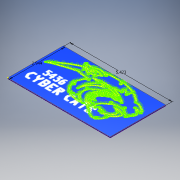
# Autodesk Inventor part: CyberCat Logo 1-27-2017
Saved by Autodesk Inventor 2016 SP2 (Build 200236200, 236)
## iProperties
Created: 2017-01-28
Part Number: CyberCat Logo 1-27-2017
Material: Generic
Document SubType Name: Modeling
Designer: CAD
Density: 1 g/cm^3
Appearance: Default
Author: CAD
Autodesk Inventor part; units mm, degrees
(part 1 of 3)
ref_plane "YZ Plane" through (0, 0, 0) normal (1, 0, 0) x (0, 1, 0)
ref_plane "XZ Plane" through (0, 0, 0) normal (0, 1, 0) x (-1, 0, 0)
ref_plane "XY Plane" through (0, 0, 0) normal (0, 0, 1) x (1, 0, 0)
sketch "Sketch5" plane through (0, 0, 0) normal (0, 1, 0) x (-1, 0, 0)
  line L0 (0, 0) -> (0, -74.7776)
  line L1 (0, -74.7776) -> (-137.7442, -74.7776)
  line L2 (-137.7442, -74.7776) -> (-137.7442, 0)
  line L3 (-137.7442, 0) -> (0, 0)
  dimension "d59" = 74.7776
  dimension "d60" = 137.7442
  constraints: 8 end point, 3 perpendicular, 1 vertical
  measures "d59" distance of L0.start L0.end
  measures "d60" distance of L0.end L1.end
extrude "Extrusion2" add sketch "Sketch5" along normal blind 0.7937
sketch "Sketch6" plane through (0, 0.7937, 0) normal (0, 1, 0) x (1, 0, 0)
  line L0 (137.7442, 74.7776) -> (0, 74.7776) projected
  line L1 (0, 74.7776) -> (137.7451, 74.7759) construction
  line L2 (137.7451, 74.7759) -> (137.7442, 0) construction
  line L3 (137.7442, 0) -> (-0.0009, 0.0017) construction
  line L4 (-0.0009, 0.0017) -> (0, 74.7776) construction
  point P0 (0, 0)
  constraints: 2 other
decal "Decal1"
sketch "Sketch7" plane through (0, 0.7937, 0) normal (0, 1, 0) x (1, 0, 0)
  circle A0 centre (6.8078, 44.1868) radius 1.651
  circle A1 centre (35.2483, 69.5859) radius 1.651
  circle A2 centre (41.5129, 60.1607) radius 1.651
  circle A3 centre (49.8624, 58.3881) radius 1.651
  circle A4 centre (44.4496, 66.9531) radius 1.651
  circle A5 centre (53.1196, 65.2289) radius 1.651
  circle A6 centre (57.1286, 60.9965) radius 1.651
  circle A7 centre (63.7205, 68.4202) radius 1.651
  circle A8 centre (83.2485, 68.8372) radius 1.651
  circle A9 centre (93.5061, 60.1607) radius 1.651
  circle A10 centre (99.5004, 60.1607) radius 1.651
  circle A11 centre (114.5732, 57.5147) radius 1.651
  circle A12 centre (130.6019, 48.3074) radius 1.651
  circle A13 centre (120.3092, 50.7732) radius 1.651
  circle A14 centre (127.1666, 41.9144) radius 1.651
  circle A15 centre (56.094, 53.7186) radius 1.651
  circle A16 centre (51.8293, 37.1588) radius 1.651
  circle A17 centre (59.035, 35.2533) radius 1.651
  circle A18 centre (64.8224, 41.5541) radius 1.651
  circle A19 centre (61.2211, 26.4773) radius 1.651
  circle A20 centre (65.5853, 26.8249) radius 1.651
  circle A21 centre (79.684, 21.2186) radius 1.651
  circle A22 centre (66.9848, 54.8596) radius 1.651
  circle A23 centre (78.8358, 51.8496) radius 1.651
  circle A24 centre (82.097, 53.5006) radius 1.651
  circle A25 centre (105.6651, 47.4221) radius 1.651
  circle A26 centre (97.355, 41.2731) radius 1.651
  circle A27 centre (84.8207, 32.3826) radius 1.651
  circle A28 centre (86.4717, 27.6903) radius 1.651
  arc A29 (94.6466, 25.5556) -> (93.8506, 25.9892) centre (95.008, 27.1666) ccw
  arc A30 (93.8506, 25.9892) -> (94.6466, 25.5556) centre (93.4892, 24.3783) ccw
  circle A31 centre (99.9904, 23.2455) radius 1.651
  circle A32 centre (104.8487, 13.4279) radius 1.651
  circle A33 centre (112.4853, 20.5125) radius 1.651
  circle A34 centre (113.5071, 44.1965) radius 1.651
  circle A35 centre (124.3721, 33.5489) radius 1.651
  line L0 (6.8078, 45.8378) -> (8.0519, 45.8378) construction
  line L1 (8.0519, 45.8378) -> (8.3576, 45.9676) construction
  line L2 (8.3576, 45.9676) -> (8.5521, 46.2871) construction
  line L3 (8.5521, 46.2871) -> (9.0107, 47.1347) construction
  line L4 (9.0107, 47.1347) -> (9.7471, 48.4269) construction
  line L5 (9.7471, 48.4269) -> (11.414, 49.9584) construction
  line L6 (11.414, 49.9584) -> (13.6061, 51.4077) construction
  line L7 (13.6061, 51.4077) -> (19.1063, 55.1419) construction
  line L8 (19.1063, 55.1419) -> (26.2805, 59.5783) construction
  line L9 (26.2805, 59.5783) -> (31.0633, 62.2885) construction
  line L10 (31.0633, 62.2885) -> (35.0489, 63.9625) construction
  line L11 (35.0489, 63.9625) -> (37.8389, 65.1565) construction
  line L12 (37.8389, 65.1565) -> (39.0415, 65.4198) construction
  line L13 (39.0415, 65.4198) -> (39.3053, 65.4198) construction
  line L14 (39.3053, 65.4198) -> (39.0576, 65.5109) construction
  line L15 (39.0576, 65.5109) -> (37.9279, 65.9163) construction
  line L16 (37.9279, 65.9163) -> (36.686, 66.5708) construction
  line L17 (36.686, 66.5708) -> (36.2832, 66.9435) construction
  line L18 (36.2832, 66.9435) -> (36.2832, 67.3428) construction
  line L19 (36.2832, 67.3428) -> (36.2832, 67.8463) construction
  line L20 (36.2832, 67.8463) -> (36.0552, 68.1455) construction
  spline S0 degree 4 poles (6.8078, 45.8378) (8.0519, 45.8378) (8.3576, 45.9676) (8.5521, 46.2871) (9.0107, 47.1347) (9.7471, 48.4269) (11.414, 49.9584) (13.6061, 51.4077) (19.1063, 55.1419) (26.2805, 59.5783) (31.0633, 62.2885) (35.0489, 63.9625) (37.8389, 65.1565) (39.0415, 65.4198) (39.3053, 65.4198) (39.0576, 65.5109) (37.9279, 65.9163) (36.686, 66.5708) (36.2832, 66.9435) (36.2832, 67.3428) (36.2832, 67.8463) (36.0552, 68.1455) knots 1 1 1 1 1 2 3 4 5 6 7 8 9 10 11 12 13 14 15 16 17 18 19 19 19 19 19
  line L21 (36.686, 70.3975) -> (37.0648, 70.1113) construction
  line L22 (37.0648, 70.1113) -> (37.624, 70.0228) construction
  line L23 (37.624, 70.0228) -> (44.0012, 70.0616) construction
  line L24 (44.0012, 70.0616) -> (44.4327, 70.1552) construction
  line L25 (44.4327, 70.1552) -> (45.8621, 70.7618) construction
  line L26 (45.8621, 70.7618) -> (47.3909, 71.4105) construction
  line L27 (47.3909, 71.4105) -> (48.4324, 71.773) construction
  line L28 (48.4324, 71.773) -> (50.9438, 72.323) construction
  line L29 (50.9438, 72.323) -> (52.679, 72.5347) construction
  line L30 (52.679, 72.5347) -> (54.742, 72.3904) construction
  line L31 (54.742, 72.3904) -> (56.914, 71.9923) construction
  line L32 (56.914, 71.9923) -> (59.3835, 71.5769) construction
  line L33 (59.3835, 71.5769) -> (60.3944, 71.3397) construction
  line L34 (60.3944, 71.3397) -> (60.7311, 71.1348) construction
  line L35 (60.7311, 71.1348) -> (60.9166, 70.9329) construction
  line L36 (60.9166, 70.9329) -> (61.1158, 71.1159) construction
  line L37 (61.1158, 71.1159) -> (61.5549, 71.5906) construction
  line L38 (61.5549, 71.5906) -> (62.519, 72.228) construction
  line L39 (62.519, 72.228) -> (63.4781, 72.438) construction
  line L40 (63.4781, 72.438) -> (65.1277, 72.438) construction
  line L41 (65.1277, 72.438) -> (65.8194, 72.7315) construction
  line L42 (65.8194, 72.7315) -> (67.0384, 72.911) construction
  line L43 (67.0384, 72.911) -> (69.9722, 73.247) construction
  line L44 (69.9722, 73.247) -> (73.1902, 73.247) construction
  line L45 (73.1902, 73.247) -> (77.615, 73.1213) construction
  line L46 (77.615, 73.1213) -> (80.8092, 73.1981) construction
  line L47 (80.8092, 73.1981) -> (81.5807, 72.9331) construction
  line L48 (81.5807, 72.9331) -> (81.9018, 72.5836) construction
  line L49 (81.9018, 72.5836) -> (81.9959, 72.1543) construction
  line L50 (81.9959, 72.1543) -> (82.3185, 72.1543) construction
  line L51 (82.3185, 72.1543) -> (82.7036, 72.2386) construction
  line L52 (82.7036, 72.2386) -> (83.0267, 72.4522) construction
  line L53 (83.0267, 72.4522) -> (83.3347, 72.7352) construction
  line L54 (83.3347, 72.7352) -> (83.6915, 72.8866) construction
  line L55 (83.6915, 72.8866) -> (84.2749, 72.8866) construction
  line L56 (84.2749, 72.8866) -> (85.5312, 72.8025) construction
  line L57 (85.5312, 72.8025) -> (86.24, 72.5421) construction
  line L58 (86.24, 72.5421) -> (87.9155, 72.4451) construction
  line L59 (87.9155, 72.4451) -> (89.2405, 72.117) construction
  line L60 (89.2405, 72.117) -> (91.2216, 71.7511) construction
  line L61 (91.2216, 71.7511) -> (93.0135, 71.3473) construction
  line L62 (93.0135, 71.3473) -> (95.8504, 70.3975) construction
  line L63 (95.8504, 70.3975) -> (99.4835, 69.2949) construction
  line L64 (99.4835, 69.2949) -> (101.2237, 68.4106) construction
  line L65 (101.2237, 68.4106) -> (101.6246, 67.8463) construction
  line L66 (101.6246, 67.8463) -> (101.6246, 67.1432) construction
  line L67 (101.6246, 67.1432) -> (101.722, 67.0838) construction
  line L68 (101.722, 67.0838) -> (102.2011, 67.3428) construction
  line L69 (102.2011, 67.3428) -> (102.836, 67.5285) construction
  line L70 (102.836, 67.5285) -> (103.6725, 67.2212) construction
  line L71 (103.6725, 67.2212) -> (105.2254, 66.4987) construction
  spline S1 degree 4 poles (36.686, 70.3975) (37.0648, 70.1113) (37.624, 70.0228) (44.0012, 70.0616) (44.4327, 70.1552) (45.8621, 70.7618) (47.3909, 71.4105) (48.4324, 71.773) (50.9438, 72.323) (52.679, 72.5347) (54.742, 72.3904) (56.914, 71.9923) (59.3835, 71.5769) (60.3944, 71.3397) (60.7311, 71.1348) (60.9166, 70.9329) (61.1158, 71.1159) (61.5549, 71.5906) (62.519, 72.228) (63.4781, 72.438) (65.1277, 72.438) (65.8194, 72.7315) (67.0384, 72.911) (69.9722, 73.247) (73.1902, 73.247) (77.615, 73.1213) (80.8092, 73.1981) (81.5807, 72.9331) (81.9018, 72.5836) (81.9959, 72.1543) (82.3185, 72.1543) (82.7036, 72.2386) (83.0267, 72.4522) (83.3347, 72.7352) (83.6915, 72.8866) (84.2749, 72.8866) (85.5312, 72.8025) (86.24, 72.5421) (87.9155, 72.4451) (89.2405, 72.117) (91.2216, 71.7511) (93.0135, 71.3473) (95.8504, 70.3975) (99.4835, 69.2949) (101.2237, 68.4106) (101.6246, 67.8463) (101.6246, 67.1432) (101.722, 67.0838) (102.2011, 67.3428) (102.836, 67.5285) (103.6725, 67.2212) (105.2254, 66.4987) knots 1 1 1 1 1 2 3 4 5 6 7 8 9 10 11 12 13 14 15 16 17 18 19 20 21 22 23 24 25 26 27 28 29 30 31 32 33 34 35 36 37 38 39 40 41 42 43 44 45 46 47 48 49 49 49 49 49
  line L72 (105.2254, 66.4987) -> (106.8582, 65.4654) construction
  line L73 (106.8582, 65.4654) -> (109.2144, 63.8128) construction
  line L74 (109.2144, 63.8128) -> (111.8392, 61.8021) construction
  line L75 (111.8392, 61.8021) -> (113.4902, 60.1511) construction
  line L76 (113.4902, 60.1511) -> (114.173, 59.4079) construction
  line L77 (114.173, 59.4079) -> (114.5732, 59.1657) construction
  spline S2 degree 4 poles (105.2254, 66.4987) (106.8582, 65.4654) (109.2144, 63.8128) (111.8392, 61.8021) (113.4902, 60.1511) (114.173, 59.4079) (114.5732, 59.1657) knots 1 1 1 1 1 2 3 4 4 4 4 4
  line L78 (116.0358, 58.2806) -> (117.3659, 58.2806) construction
  line L79 (117.3659, 58.2806) -> (118.6414, 58.2806) construction
  line L80 (118.6414, 58.2806) -> (120.0673, 58.055) construction
  line L81 (120.0673, 58.055) -> (122.3159, 57.0087) construction
  line L82 (122.3159, 57.0087) -> (126.3877, 54.85) construction
  line L83 (126.3877, 54.85) -> (129.1696, 52.4145) construction
  line L84 (129.1696, 52.4145) -> (130.2329, 50.885) construction
  line L85 (130.2329, 50.885) -> (130.5445, 50.4137) construction
  line L86 (130.5445, 50.4137) -> (130.7761, 50.0633) construction
  line L87 (130.7761, 50.0633) -> (130.8588, 49.9383) construction
  spline S3 degree 4 poles (116.0358, 58.2806) (117.3659, 58.2806) (118.6414, 58.2806) (120.0673, 58.055) (122.3159, 57.0087) (126.3877, 54.85) (129.1696, 52.4145) (130.2329, 50.885) (130.5445, 50.4137) (130.7761, 50.0633) (130.8588, 49.9383) knots 1 1 1 1 1 2 3 4 5 6 7 8 8 8 8 8
  circle A36 centre (6.8078, 44.1868) radius 0.889
  circle A37 centre (41.5129, 60.1607) radius 0.889
  circle A38 centre (44.4496, 66.9531) radius 0.889
  circle A39 centre (53.1196, 65.2289) radius 0.889
  circle A40 centre (57.1286, 60.9965) radius 0.889
  circle A41 centre (56.094, 53.7186) radius 0.889
  circle A42 centre (51.8293, 37.1588) radius 0.889
  circle A43 centre (59.035, 35.2533) radius 0.889
  circle A44 centre (61.2211, 26.4773) radius 0.889
  circle A45 centre (64.8224, 41.5541) radius 0.889
  circle A46 centre (66.9848, 54.8596) radius 0.889
  circle A47 centre (63.7205, 68.4202) radius 0.889
  circle A48 centre (35.2483, 69.5859) radius 0.889
  circle A49 centre (49.8624, 58.3881) radius 0.889
  circle A50 centre (82.097, 53.5006) radius 0.889
  circle A51 centre (78.8358, 51.8496) radius 0.889
  circle A52 centre (65.5853, 26.8249) radius 0.889
  circle A53 centre (79.684, 21.2186) radius 0.889
  circle A54 centre (86.4717, 27.6903) radius 0.889
  circle A55 centre (84.8207, 32.3826) radius 0.889
  circle A56 centre (95.008, 27.1666) radius 0.889
  circle A57 centre (93.4892, 24.3783) radius 0.889
  circle A58 centre (97.355, 41.2731) radius 0.889
  circle A59 centre (105.6651, 47.4221) radius 0.889
  circle A60 centre (93.5061, 60.1607) radius 0.889
  circle A61 centre (99.5004, 60.1607) radius 0.889
  circle A62 centre (114.5732, 57.5147) radius 0.889
  circle A63 centre (120.3092, 50.7732) radius 0.889
  circle A64 centre (127.1666, 41.9144) radius 0.889
  circle A65 centre (130.6019, 48.3074) radius 0.889
  circle A66 centre (124.3721, 33.5489) radius 0.889
  circle A67 centre (113.5071, 44.1965) radius 0.889
  circle A68 centre (104.8487, 13.4279) radius 0.889
  circle A69 centre (99.9904, 23.2455) radius 0.889
  circle A70 centre (112.4853, 20.5125) radius 0.889
  line L88 (129.3056, 47.285) -> (128.6834, 47.6216) construction
  line L89 (128.6834, 47.6216) -> (128.2041, 47.9133) construction
  line L90 (128.2041, 47.9133) -> (127.6309, 47.9133) construction
  line L91 (127.6309, 47.9133) -> (127.6309, 47.7021) construction
  line L92 (127.6309, 47.7021) -> (127.6309, 47.4374) construction
  line L93 (127.6309, 47.4374) -> (128.0384, 47.0641) construction
  line L94 (128.0384, 47.0641) -> (128.6987, 46.4533) construction
  line L95 (128.6987, 46.4533) -> (129.7126, 45.5394) construction
  line L96 (129.7126, 45.5394) -> (130.305, 44.6433) construction
  line L97 (130.305, 44.6433) -> (130.7259, 43.2144) construction
  line L98 (130.7259, 43.2144) -> (130.6016, 41.631) construction
  line L99 (130.6016, 41.631) -> (129.9774, 39.9124) construction
  line L100 (129.9774, 39.9124) -> (129.7126, 39.4529) construction
  line L101 (129.7126, 39.4529) -> (129.0373, 38.7229) construction
  line L102 (129.0373, 38.7229) -> (128.1187, 37.7299) construction
  line L103 (128.1187, 37.7299) -> (127.4807, 37.0403) construction
  line L104 (127.4807, 37.0403) -> (127.1494, 36.4595) construction
  line L105 (127.1494, 36.4595) -> (127.1494, 35.2254) construction
  line L106 (127.1494, 35.2254) -> (127.0463, 34.574) construction
  line L107 (127.0463, 34.574) -> (126.4766, 34.0429) construction
  line L108 (126.4766, 34.0429) -> (126.2604, 33.6116) construction
  line L109 (126.2604, 33.6116) -> (125.9704, 33.1353) construction
  spline S4 degree 4 poles (129.3056, 47.285) (128.6834, 47.6216) (128.2041, 47.9133) (127.6309, 47.9133) (127.6309, 47.7021) (127.6309, 47.4374) (128.0384, 47.0641) (128.6987, 46.4533) (129.7126, 45.5394) (130.305, 44.6433) (130.7259, 43.2144) (130.6016, 41.631) (129.9774, 39.9124) (129.7126, 39.4529) (129.0373, 38.7229) (128.1187, 37.7299) (127.4807, 37.0403) (127.1494, 36.4595) (127.1494, 35.2254) (127.0463, 34.574) (126.4766, 34.0429) (126.2604, 33.6116) (125.9704, 33.1353) knots 1 1 1 1 1 2 3 4 5 6 7 8 9 10 11 12 13 14 15 16 17 18 19 20 20 20 20 20
  line L110 (122.796, 34.0405) -> (122.546, 34.4186) construction
  line L111 (122.546, 34.4186) -> (121.9434, 34.9796) construction
  line L112 (121.9434, 34.9796) -> (121.2954, 35.4818) construction
  line L113 (121.2954, 35.4818) -> (120.7411, 35.9945) construction
  line L114 (120.7411, 35.9945) -> (120.0673, 36.499) construction
  line L115 (120.0673, 36.499) -> (119.5784, 36.7966) construction
  line L116 (119.5784, 36.7966) -> (118.8662, 37.1468) construction
  line L117 (118.8662, 37.1468) -> (118.1515, 37.6752) construction
  line L118 (118.1515, 37.6752) -> (117.513, 37.9954) construction
  line L119 (117.513, 37.9954) -> (116.4961, 38.6144) construction
  line L120 (116.4961, 38.6144) -> (115.2293, 39.0855) construction
  line L121 (115.2293, 39.0855) -> (114.5732, 39.0855) construction
  line L122 (114.5732, 39.0855) -> (114.1479, 39.91) construction
  line L123 (114.1479, 39.91) -> (113.7598, 40.5655) construction
  line L124 (113.7598, 40.5655) -> (113.5786, 40.8396) construction
  line L125 (113.5786, 40.8396) -> (113.4566, 40.653) construction
  line L126 (113.4566, 40.653) -> (113.2805, 40.3636) construction
  line L127 (113.2805, 40.3636) -> (112.7385, 40.175) construction
  line L128 (112.7385, 40.175) -> (111.5844, 40.175) construction
  line L129 (111.5844, 40.175) -> (110.1447, 40.175) construction
  line L130 (110.1447, 40.175) -> (108.9041, 40.175) construction
  line L131 (108.9041, 40.175) -> (107.0369, 40.175) construction
  line L132 (107.0369, 40.175) -> (105.6482, 39.91) construction
  line L133 (105.6482, 39.91) -> (103.6725, 39.3406) construction
  line L134 (103.6725, 39.3406) -> (102.1495, 39.0855) construction
  line L135 (102.1495, 39.0855) -> (101.1345, 39.0855) construction
  line L136 (101.1345, 39.0855) -> (101.0047, 38.9663) construction
  line L137 (101.0047, 38.9663) -> (101.0493, 38.6006) construction
  line L138 (101.0493, 38.6006) -> (100.9043, 38.224) construction
  line L139 (100.9043, 38.224) -> (99.0745, 36.6349) construction
  line L140 (99.0745, 36.6349) -> (97.3379, 35.2602) construction
  line L141 (97.3379, 35.2602) -> (95.9794, 34.306) construction
  line L142 (95.9794, 34.306) -> (94.4909, 33.1329) construction
  line L143 (94.4909, 33.1329) -> (93.4892, 32.0282) construction
  line L144 (93.4892, 32.0282) -> (91.9786, 30.3953) construction
  line L145 (91.9786, 30.3953) -> (91.3738, 29.3292) construction
  line L146 (91.3738, 29.3292) -> (91.051, 28.7602) construction
  line L147 (91.051, 28.7602) -> (90.7428, 27.5702) construction
  line L148 (90.7428, 27.5702) -> (90.7428, 27.8795) construction
  line L149 (90.7428, 27.8795) -> (91.2216, 26.2776) construction
  line L150 (91.2216, 26.2776) -> (91.8382, 25.9235) construction
  line L151 (91.8382, 25.9235) -> (92.1175, 25.9235) construction
  line L152 (92.1175, 25.9235) -> (93.3559, 26.0239) construction
  spline S5 degree 4 poles (122.796, 34.0405) (122.546, 34.4186) (121.9434, 34.9796) (121.2954, 35.4818) (120.7411, 35.9945) (120.0673, 36.499) (119.5784, 36.7966) (118.8662, 37.1468) (118.1515, 37.6752) (117.513, 37.9954) (116.4961, 38.6144) (115.2293, 39.0855) (114.5732, 39.0855) (114.1479, 39.91) (113.7598, 40.5655) (113.5786, 40.8396) (113.4566, 40.653) (113.2805, 40.3636) (112.7385, 40.175) (111.5844, 40.175) (110.1447, 40.175) (108.9041, 40.175) (107.0369, 40.175) (105.6482, 39.91) (103.6725, 39.3406) (102.1495, 39.0855) (101.1345, 39.0855) (101.0047, 38.9663) (101.0493, 38.6006) (100.9043, 38.224) (99.0745, 36.6349) (97.3379, 35.2602) (95.9794, 34.306) (94.4909, 33.1329) (93.4892, 32.0282) (91.9786, 30.3953) (91.3738, 29.3292) (91.051, 28.7602) (90.7428, 27.5702) (90.7428, 27.8795) (91.2216, 26.2776) (91.8382, 25.9235) (92.1175, 25.9235) (93.3559, 26.0239) knots 1 1 1 1 1 2 3 4 5 6 7 8 9 10 11 12 13 14 15 16 17 18 19 20 21 22 23 24 25 26 27 28 29 30 31 32 33 34 35 36 37 38 39 40 41 41 41 41 41
  line L153 (96.5618, 27.7248) -> (97.1191, 27.3038) construction
  line L154 (97.1191, 27.3038) -> (97.3379, 27.0555) construction
  line L155 (97.3379, 27.0555) -> (97.8653, 27.0555) construction
  line L156 (97.8653, 27.0555) -> (99.2208, 26.9607) construction
  line L157 (99.2208, 26.9607) -> (100.4553, 26.8744) construction
  line L158 (100.4553, 26.8744) -> (102.4187, 26.5825) construction
  line L159 (102.4187, 26.5825) -> (103.8312, 26.2776) construction
  line L160 (103.8312, 26.2776) -> (105.8325, 25.1736) construction
  line L161 (105.8325, 25.1736) -> (106.8582, 24.7571) construction
  line L162 (106.8582, 24.7571) -> (107.2071, 24.5771) construction
  line L163 (107.2071, 24.5771) -> (107.5617, 24.7071) construction
  line L164 (107.5617, 24.7071) -> (108.6368, 25.429) construction
  line L165 (108.6368, 25.429) -> (109.6035, 26.2607) construction
  line L166 (109.6035, 26.2607) -> (110.7834, 27.3596) construction
  line L167 (110.7834, 27.3596) -> (112.2266, 28.4756) construction
  line L168 (112.2266, 28.4756) -> (113.2514, 29.5529) construction
  line L169 (113.2514, 29.5529) -> (113.6692, 30.3296) construction
  line L170 (113.6692, 30.3296) -> (113.9538, 31.1767) construction
  line L171 (113.9538, 31.1767) -> (113.8316, 31.8979) construction
  line L172 (113.8316, 31.8979) -> (113.6692, 32.5806) construction
  line L173 (113.6692, 32.5806) -> (112.8943, 33.1329) construction
  line L174 (112.8943, 33.1329) -> (111.8392, 33.9603) construction
  line L175 (111.8392, 33.9603) -> (110.5103, 34.7416) construction
  line L176 (110.5103, 34.7416) -> (109.2144, 35.4568) construction
  line L177 (109.2144, 35.4568) -> (107.8042, 36.1539) construction
  line L178 (107.8042, 36.1539) -> (106.5991, 36.7966) construction
  line L179 (106.5991, 36.7966) -> (105.8073, 37.2918) construction
  line L180 (105.8073, 37.2918) -> (105.8439, 37.8155) construction
  line L181 (105.8439, 37.8155) -> (106.2177, 38.1002) construction
  line L182 (106.2177, 38.1002) -> (106.8359, 38.1503) construction
  line L183 (106.8359, 38.1503) -> (107.3161, 38.6006) construction
  line L184 (107.3161, 38.6006) -> (108.4314, 38.6006) construction
  line L185 (108.4314, 38.6006) -> (110.2731, 38.6006) construction
  line L186 (110.2731, 38.6006) -> (110.9494, 38.6006) construction
  line L187 (110.9494, 38.6006) -> (112.4421, 38.141) construction
  line L188 (112.4421, 38.141) -> (115.6268, 37.5536) construction
  line L189 (115.6268, 37.5536) -> (119.6082, 36.1285) construction
  line L190 (119.6082, 36.1285) -> (120.6634, 34.3509) construction
  line L191 (120.6634, 34.3509) -> (121.6789, 32.8567) construction
  line L192 (121.6789, 32.8567) -> (121.1711, 31.5373) construction
  line L193 (121.1711, 31.5373) -> (121.1711, 31.2475) construction
  line L194 (121.1711, 31.2475) -> (120.0032, 29.2997) construction
  line L195 (120.0032, 29.2997) -> (118.8405, 27.3284) construction
  line L196 (118.8405, 27.3284) -> (116.5079, 25.429) construction
  line L197 (116.5079, 25.429) -> (114.7457, 23.7264) construction
  spline S6 degree 4 poles (96.5618, 27.7248) (97.1191, 27.3038) (97.3379, 27.0555) (97.8653, 27.0555) (99.2208, 26.9607) (100.4553, 26.8744) (102.4187, 26.5825) (103.8312, 26.2776) (105.8325, 25.1736) (106.8582, 24.7571) (107.2071, 24.5771) (107.5617, 24.7071) (108.6368, 25.429) (109.6035, 26.2607) (110.7834, 27.3596) (112.2266, 28.4756) (113.2514, 29.5529) (113.6692, 30.3296) (113.9538, 31.1767) (113.8316, 31.8979) (113.6692, 32.5806) (112.8943, 33.1329) (111.8392, 33.9603) (110.5103, 34.7416) (109.2144, 35.4568) (107.8042, 36.1539) (106.5991, 36.7966) (105.8073, 37.2918) (105.8439, 37.8155) (106.2177, 38.1002) (106.8359, 38.1503) (107.3161, 38.6006) (108.4314, 38.6006) (110.2731, 38.6006) (110.9494, 38.6006) (112.4421, 38.141) (115.6268, 37.5536) (119.6082, 36.1285) (120.6634, 34.3509) (121.6789, 32.8567) (121.1711, 31.5373) (121.1711, 31.2475) (120.0032, 29.2997) (118.8405, 27.3284) (116.5079, 25.429) (114.7457, 23.7264) (113.5658, 22.5866) (113.5658, 21.9145) (113.4584, 21.8462) knots 1 1 1 1 1 2 3 4 5 6 7 8 9 10 11 12 13 14 15 16 17 18 19 20 21 22 23 24 25 26 27 28 29 30 31 32 33 34 35 36 37 38 39 40 41 42 43 44 45 45.458778 45.458778 45.458778 45.458778 45.458778
  line L198 (114.7457, 23.7264) -> (113.5658, 22.5866) construction
  line L199 (113.5658, 22.5866) -> (113.5658, 21.9145) construction
  line L200 (113.5658, 21.9145) -> (113.4584, 21.8462) construction
  line L201 (113.3278, 19.0927) -> (112.8311, 18.6364) construction
  line L202 (112.8311, 18.6364) -> (112.3668, 17.3485) construction
  line L203 (112.3668, 17.3485) -> (111.9634, 16.088) construction
  line L204 (111.9634, 16.088) -> (111.333, 15.2536) construction
  line L205 (111.333, 15.2536) -> (110.2619, 13.4817) construction
  line L206 (110.2619, 13.4817) -> (109.3991, 12.3078) construction
  line L207 (109.3991, 12.3078) -> (109.1201, 12.1294) construction
  line L208 (109.1201, 12.1294) -> (108.7461, 12.2171) construction
  line L209 (108.7461, 12.2171) -> (108.2453, 12.2171) construction
  line L210 (108.2453, 12.2171) -> (108.1253, 11.7053) construction
  line L211 (108.1253, 11.7053) -> (107.9865, 11.1137) construction
  line L212 (107.9865, 11.1137) -> (107.2305, 10.4191) construction
  line L213 (107.2305, 10.4191) -> (106.373, 10.2313) construction
  line L214 (106.373, 10.2313) -> (105.6482, 10.1717) construction
  line L215 (105.6482, 10.1717) -> (104.1946, 10.0539) construction
  line L216 (104.1946, 10.0539) -> (102.4659, 10.103) construction
  line L217 (102.4659, 10.103) -> (101.4881, 10.2777) construction
  line L218 (101.4881, 10.2777) -> (101.0696, 10.6634) construction
  line L219 (101.0696, 10.6634) -> (100.0866, 10.896) construction
  line L220 (100.0866, 10.896) -> (99.1123, 11.2646) construction
  line L221 (99.1123, 11.2646) -> (98.4073, 11.8091) construction
  line L222 (98.4073, 11.8091) -> (97.6669, 12.0988) construction
  line L223 (97.6669, 12.0988) -> (96.6293, 12.4903) construction
  line L224 (96.6293, 12.4903) -> (94.1378, 13.4279) construction
  line L225 (94.1378, 13.4279) -> (92.913, 14.5562) construction
  line L226 (92.913, 14.5562) -> (91.6762, 15.9378) construction
  line L227 (91.6762, 15.9378) -> (90.4166, 17.3088) construction
  line L228 (90.4166, 17.3088) -> (89.317, 17.8828) construction
  line L229 (89.317, 17.8828) -> (87.5364, 18.8615) construction
  line L230 (87.5364, 18.8615) -> (85.179, 20.1703) construction
  line L231 (85.179, 20.1703) -> (79.684, 23.9515) construction
  line L232 (79.684, 23.9515) -> (78.4367, 24.8965) construction
  line L233 (78.4367, 24.8965) -> (76.6314, 26.8744) construction
  line L234 (76.6314, 26.8744) -> (75.4186, 28.4756) construction
  line L235 (75.4186, 28.4756) -> (74.0816, 30.498) construction
  line L236 (74.0816, 30.498) -> (72.8695, 32.3314) construction
  line L237 (72.8695, 32.3314) -> (72.5719, 33.3735) construction
  line L238 (72.5719, 33.3735) -> (72.414, 34.6991) construction
  line L239 (72.414, 34.6991) -> (72.414, 35.5831) construction
  line L240 (72.414, 35.5831) -> (72.414, 36.7499) construction
  line L241 (72.414, 36.7499) -> (72.414, 37.9579) construction
  line L242 (72.414, 37.9579) -> (72.5871, 39.3869) construction
  line L243 (72.5871, 39.3869) -> (72.9956, 40.393) construction
  line L244 (72.9956, 40.393) -> (73.4331, 41.5541) construction
  line L245 (73.4331, 41.5541) -> (74.1548, 42.8881) construction
  line L246 (74.1548, 42.8881) -> (74.9232, 43.9288) construction
  line L247 (74.9232, 43.9288) -> (75.7453, 44.6842) construction
  line L248 (75.7453, 44.6842) -> (76.7373, 45.5957) construction
  line L249 (76.7373, 45.5957) -> (77.896, 46.4533) construction
  line L250 (77.896, 46.4533) -> (79.5586, 47.5697) construction
  line L251 (79.5586, 47.5697) -> (81.5975, 48.5492) construction
  line L252 (81.5975, 48.5492) -> (83.2485, 49.2482) construction
  line L253 (83.2485, 49.2482) -> (84.923, 49.7857) construction
  line L254 (84.923, 49.7857) -> (87.5822, 50.0633) construction
  line L255 (87.5822, 50.0633) -> (88.9622, 50.4137) construction
  line L256 (88.9622, 50.4137) -> (90.2435, 50.4137) construction
  line L257 (90.2435, 50.4137) -> (93.0912, 50.241) construction
  line L258 (93.0912, 50.241) -> (95.5429, 50.0008) construction
  line L259 (95.5429, 50.0008) -> (97.7737, 50.0008) construction
  line L260 (97.7737, 50.0008) -> (99.3555, 50.0008) construction
  line L261 (99.3555, 50.0008) -> (99.7029, 49.6407) construction
  line L262 (99.7029, 49.6407) -> (100.1413, 49.3543) construction
  line L263 (100.1413, 49.3543) -> (100.9768, 49.3543) construction
  line L264 (100.9768, 49.3543) -> (101.2237, 49.411) construction
  line L265 (101.2237, 49.411) -> (101.2237, 49.5355) construction
  line L266 (101.2237, 49.5355) -> (101.0573, 49.6612) construction
  line L267 (101.0573, 49.6612) -> (100.6615, 50.092) construction
  line L268 (100.6615, 50.092) -> (100.0705, 50.3802) construction
  line L269 (100.0705, 50.3802) -> (100.0705, 50.6494) construction
  line L270 (100.0705, 50.6494) -> (99.4103, 51.0143) construction
  line L271 (99.4103, 51.0143) -> (98.4862, 51.4839) construction
  line L272 (98.4862, 51.4839) -> (98.0805, 51.7905) construction
  line L273 (98.0805, 51.7905) -> (97.977, 51.9469) construction
  line L274 (97.977, 51.9469) -> (97.904, 51.9469) construction
  line L275 (97.904, 51.9469) -> (97.8494, 51.8903) construction
  line L276 (97.8494, 51.8903) -> (97.7867, 51.4941) construction
  line L277 (97.7867, 51.4941) -> (97.7246, 50.9606) construction
  line L278 (97.7246, 50.9606) -> (97.6392, 50.7994) construction
  line L279 (97.6392, 50.7994) -> (97.3379, 50.7353) construction
  line L280 (97.3379, 50.7353) -> (96.7646, 50.7353) construction
  line L281 (96.7646, 50.7353) -> (95.7613, 50.7353) construction
  line L282 (95.7613, 50.7353) -> (94.3782, 50.832) construction
  line L283 (94.3782, 50.832) -> (92.6343, 50.832) construction
  line L284 (92.6343, 50.832) -> (90.8825, 50.832) construction
  line L285 (90.8825, 50.832) -> (89.8038, 50.832) construction
  line L286 (89.8038, 50.832) -> (88.0639, 50.832) construction
  line L287 (88.0639, 50.832) -> (86.889, 50.6494) construction
  line L288 (86.889, 50.6494) -> (85.5827, 50.3508) construction
  line L289 (85.5827, 50.3508) -> (82.8652, 49.7866) construction
  line L290 (82.8652, 49.7866) -> (81.208, 49.1964) construction
  line L291 (81.208, 49.1964) -> (80.573, 49.1964) construction
  line L292 (80.573, 49.1964) -> (79.9721, 48.6442) construction
  line L293 (79.9721, 48.6442) -> (78.795, 48.0849) construction
  line L294 (78.795, 48.0849) -> (77.3293, 47.3783) construction
  line L295 (77.3293, 47.3783) -> (75.5676, 46.3352) construction
  line L296 (75.5676, 46.3352) -> (74.2286, 45.45) construction
  line L297 (74.2286, 45.45) -> (72.9727, 44.477) construction
  line L298 (72.9727, 44.477) -> (72.3611, 44.0637) construction
  line L299 (72.3611, 44.0637) -> (71.8015, 43.5654) construction
  line L300 (71.8015, 43.5654) -> (70.955, 42.8034) construction
  line L301 (70.955, 42.8034) -> (70.2736, 42.2842) construction
  line L302 (70.2736, 42.2842) -> (69.4879, 41.5541) construction
  line L303 (69.4879, 41.5541) -> (69.1376, 41.2322) construction
  line L304 (69.1376, 41.2322) -> (68.7935, 41.2322) construction
  line L305 (68.7935, 41.2322) -> (68.6358, 41.0834) construction
  line L306 (68.6358, 41.0834) -> (68.5546, 40.7463) construction
  line L307 (68.5546, 40.7463) -> (68.3854, 39.8233) construction
  line L308 (68.3854, 39.8233) -> (68.0417, 39.4977) construction
  line L309 (68.0417, 39.4977) -> (67.4182, 38.141) construction
  line L310 (67.4182, 38.141) -> (66.8809, 36.6349) construction
  line L311 (66.8809, 36.6349) -> (66.8809, 35.0992) construction
  line L312 (66.8809, 35.0992) -> (66.9848, 33.2764) construction
  line L313 (66.9848, 33.2764) -> (67.2562, 32.0282) construction
  line L314 (67.2562, 32.0282) -> (67.4232, 31.2475) construction
  line L315 (67.4232, 31.2475) -> (67.4948, 30.9206) construction
  line L316 (67.4948, 30.9206) -> (67.4226, 29.8877) construction
  line L317 (67.4226, 29.8877) -> (67.7636, 29.8877) construction
  line L318 (67.7636, 29.8877) -> (68.7453, 29.275) construction
  line L319 (68.7453, 29.275) -> (69.5339, 28.1652) construction
  line L320 (69.5339, 28.1652) -> (71.5457, 26.1535) construction
  line L321 (71.5457, 26.1535) -> (72.7703, 25.1478) construction
  line L322 (72.7703, 25.1478) -> (73.5314, 24.5777) construction
  line L323 (73.5314, 24.5777) -> (74.6879, 24.0396) construction
  line L324 (74.6879, 24.0396) -> (75.5659, 23.5117) construction
  line L325 (75.5659, 23.5117) -> (76.3924, 23.3477) construction
  line L326 (76.3924, 23.3477) -> (77.1848, 22.8696) construction
  line L327 (77.1848, 22.8696) -> (78.361, 22.8696) construction
  line L328 (78.361, 22.8696) -> (79.684, 22.8696) construction
  spline S7 degree 4 number of poles 129
  line L329 (67.1583, 27.3265) -> (67.278, 27.4116) construction
  line L330 (67.278, 27.4116) -> (67.5072, 27.4116) construction
  line L331 (67.5072, 27.4116) -> (68.0428, 26.8249) construction
  line L332 (68.0428, 26.8249) -> (69.383, 25.3662) construction
  line L333 (69.383, 25.3662) -> (70.7406, 24.309) construction
  line L334 (70.7406, 24.309) -> (71.9962, 23.3481) construction
  line L335 (71.9962, 23.3481) -> (74.5761, 22.3568) construction
  line L336 (74.5761, 22.3568) -> (74.5761, 22.0615) construction
  line L337 (74.5761, 22.0615) -> (74.5761, 21.761) construction
  line L338 (74.5761, 21.761) -> (73.9732, 21.6063) construction
  line L339 (73.9732, 21.6063) -> (72.804, 21.5679) construction
  line L340 (72.804, 21.5679) -> (71.6804, 21.6432) construction
  line L341 (71.6804, 21.6432) -> (70.6241, 21.9748) construction
  line L342 (70.6241, 21.9748) -> (68.7935, 21.9748) construction
  line L343 (68.7935, 21.9748) -> (67.1781, 22.2342) construction
  line L344 (67.1781, 22.2342) -> (65.1042, 22.7712) construction
  line L345 (65.1042, 22.7712) -> (63.1714, 23.4297) construction
  line L346 (63.1714, 23.4297) -> (61.924, 23.888) construction
  line L347 (61.924, 23.888) -> (61.4732, 24.0396) construction
  line L348 (61.4732, 24.0396) -> (61.1158, 24.1677) construction
  line L349 (61.1158, 24.1677) -> (60.8239, 24.424) construction
  line L350 (60.8239, 24.424) -> (60.8239, 24.6421) construction
  line L351 (60.8239, 24.6421) -> (60.8239, 24.789) construction
  line L352 (60.8239, 24.789) -> (60.9433, 24.8223) construction
  spline S8 degree 4 poles (67.1583, 27.3265) (67.278, 27.4116) (67.5072, 27.4116) (68.0428, 26.8249) (69.383, 25.3662) (70.7406, 24.309) (71.9962, 23.3481) (74.5761, 22.3568) (74.5761, 22.0615) (74.5761, 21.761) (73.9732, 21.6063) (72.804, 21.5679) (71.6804, 21.6432) (70.6241, 21.9748) (68.7935, 21.9748) (67.1781, 22.2342) (65.1042, 22.7712) (63.1714, 23.4297) (61.924, 23.888) (61.4732, 24.0396) (61.1158, 24.1677) (60.8239, 24.424) (60.8239, 24.6421) (60.8239, 24.789) (60.9433, 24.8223) knots 0 0 0 0 0 1 2 3 4 5 6 7 8 9 10 11 12 13 14 15 16 17 18 19 20 21 21 21 21 21
  line L353 (60.9433, 24.8223) -> (60.9971, 24.8415)
  line L354 (59.711, 27.1448) -> (58.9816, 26.7139) construction
  line L355 (58.9816, 26.7139) -> (58.3088, 26.4155) construction
  line L356 (58.3088, 26.4155) -> (57.8131, 26.4155) construction
  line L357 (57.8131, 26.4155) -> (57.2498, 26.4155) construction
  line L358 (57.2498, 26.4155) -> (56.6134, 26.8103) construction
  line L359 (56.6134, 26.8103) -> (55.5125, 27.6757) construction
  line L360 (55.5125, 27.6757) -> (54.5273, 28.7055) construction
  line L361 (54.5273, 28.7055) -> (53.9435, 29.6016) construction
  line L362 (53.9435, 29.6016) -> (53.3366, 30.2591) construction
  line L363 (53.3366, 30.2591) -> (52.6255, 31.3261) construction
  line L364 (52.6255, 31.3261) -> (52.1081, 31.8834) construction
  line L365 (52.1081, 31.8834) -> (51.6582, 32.7263) construction
  line L366 (51.6582, 32.7263) -> (51.3783, 33.1183) construction
  line L367 (51.3783, 33.1183) -> (51.0673, 33.851) construction
  line L368 (51.0673, 33.851) -> (50.7785, 34.5317) construction
  line L369 (50.7785, 34.5317) -> (50.6341, 34.965) construction
  line L370 (50.6341, 34.965) -> (50.4886, 35.3859) construction
  line L371 (50.4886, 35.3859) -> (50.4886, 35.9261) construction
  line L372 (50.4886, 35.9261) -> (50.3306, 36.0754) construction
  spline S9 degree 4 poles (59.711, 27.1448) (58.9816, 26.7139) (58.3088, 26.4155) (57.8131, 26.4155) (57.2498, 26.4155) (56.6134, 26.8103) (55.5125, 27.6757) (54.5273, 28.7055) (53.9435, 29.6016) (53.3366, 30.2591) (52.6255, 31.3261) (52.1081, 31.8834) (51.6582, 32.7263) (51.3783, 33.1183) (51.0673, 33.851) (50.7785, 34.5317) (50.6341, 34.965) (50.4886, 35.3859) (50.4886, 35.9261) (50.3306, 36.0754) knots 0 0 0 0 0 1 2 3 4 5 6 7 8 9 10 11 12 13 14 15 16 16 16 16 16
  line L373 (50.3306, 36.0754) -> (50.1783, 36.283) construction
  line L374 (50.1783, 36.283) -> (50.0663, 36.7966) construction
  line L375 (50.0663, 36.7966) -> (50.0663, 36.9997) construction
  line L376 (50.0663, 36.9997) -> (50.0921, 37.1588) construction
  spline S10 degree 4 poles (50.3306, 36.0754) (50.1783, 36.283) (50.0663, 36.7966) (50.0663, 36.9997) (50.0921, 37.1588) knots 1 1 1 1 1 2 2 2 2 2
  arc A71 (50.1882, 37.3395) -> (50.0921, 37.1588) centre (50.5947, 37.0072) ccw
  line L377 (52.6873, 38.5693) -> (51.6883, 39.3406) construction
  line L378 (51.6883, 39.3406) -> (51.2905, 39.3701) construction
  line L379 (51.2905, 39.3701) -> (50.9983, 39.6826) construction
  line L380 (50.9983, 39.6826) -> (50.3306, 40.2026) construction
  line L381 (50.3306, 40.2026) -> (50.065, 40.5083) construction
  line L382 (50.065, 40.5083) -> (50.0218, 41.0834) construction
  line L383 (50.0218, 41.0834) -> (50.0218, 41.6686) construction
  line L384 (50.0218, 41.6686) -> (49.9708, 41.722) construction
  line L385 (49.9708, 41.722) -> (50.4886, 42.8987) construction
  line L386 (50.4886, 42.8987) -> (50.7785, 43.6237) construction
  line L387 (50.7785, 43.6237) -> (51.2905, 44.9045) construction
  line L388 (51.2905, 44.9045) -> (52.4791, 47.3783) construction
  line L389 (52.4791, 47.3783) -> (52.9811, 48.6442) construction
  line L390 (52.9811, 48.6442) -> (53.9435, 49.8766) construction
  line L391 (53.9435, 49.8766) -> (54.5273, 50.6756) construction
  line L392 (54.5273, 50.6756) -> (55.6003, 50.7732) construction
  line L393 (55.6003, 50.7732) -> (57.1286, 50.7732) construction
  line L394 (57.1286, 50.7732) -> (57.6313, 50.832) construction
  line L395 (57.6313, 50.832) -> (57.7728, 51.2273) construction
  line L396 (57.7728, 51.2273) -> (57.7728, 52.0956) construction
  line L397 (57.7728, 52.0956) -> (57.6442, 53.1506) construction
  spline S11 degree 4 poles (52.6873, 38.5693) (51.6883, 39.3406) (51.2905, 39.3701) (50.9983, 39.6826) (50.3306, 40.2026) (50.065, 40.5083) (50.0218, 41.0834) (50.0218, 41.6686) (49.9708, 41.722) (50.4886, 42.8987) (50.7785, 43.6237) (51.2905, 44.9045) (52.4791, 47.3783) (52.9811, 48.6442) (53.9435, 49.8766) (54.5273, 50.6756) (55.6003, 50.7732) (57.1286, 50.7732) (57.6313, 50.832) (57.7728, 51.2273) (57.7728, 52.0956) (57.6442, 53.1506) knots 1 1 1 1 1 2 3 4 5 6 7 8 9 10 11 12 13 14 15 16 17 18 19 19 19 19 19
  line L398 (54.9007, 54.8596) -> (54.4765, 54.7136) construction
  line L399 (54.4765, 54.7136) -> (53.9435, 54.7136) construction
  line L400 (53.9435, 54.7136) -> (52.7301, 54.7136) construction
  line L401 (52.7301, 54.7136) -> (51.4894, 54.7136) construction
  line L402 (51.4894, 54.7136) -> (49.6881, 54.7136) construction
  line L403 (49.6881, 54.7136) -> (47.5629, 54.8596) construction
  line L404 (47.5629, 54.8596) -> (45.9313, 55.1419) construction
  line L405 (45.9313, 55.1419) -> (43.8712, 55.2718) construction
  line L406 (43.8712, 55.2718) -> (43.2767, 55.3696) construction
  line L407 (43.2767, 55.3696) -> (42.8621, 55.6655) construction
  line L408 (42.8621, 55.6655) -> (41.1619, 56.0816) construction
  line L409 (41.1619, 56.0816) -> (40.5893, 56.292) construction
  line L410 (40.5893, 56.292) -> (39.9821, 56.292) construction
  line L411 (39.9821, 56.292) -> (39.2171, 56.292) construction
  line L412 (39.2171, 56.292) -> (38.4402, 56.0817) construction
  line L413 (38.4402, 56.0817) -> (37.6861, 55.8637) construction
  line L414 (37.6861, 55.8637) -> (36.3853, 55.5789) construction
  line L415 (36.3853, 55.5789) -> (36.1116, 55.3696) construction
  line L416 (36.1116, 55.3696) -> (35.3358, 55.1419) construction
  line L417 (35.3358, 55.1419) -> (34.2482, 54.9037) construction
  line L418 (34.2482, 54.9037) -> (32.1688, 54.4484) construction
  line L419 (32.1688, 54.4484) -> (30.0993, 53.784) construction
  line L420 (30.0993, 53.784) -> (28.8674, 53.4238) construction
  line L421 (28.8674, 53.4238) -> (27.2155, 52.8935) construction
  line L422 (27.2155, 52.8935) -> (25.7568, 52.4669) construction
  line L423 (25.7568, 52.4669) -> (23.2013, 51.5305) construction
  line L424 (23.2013, 51.5305) -> (21.9891, 51.1414) construction
  line L425 (21.9891, 51.1414) -> (20.9902, 50.832) construction
  line L426 (20.9902, 50.832) -> (19.4801, 50.2361) construction
  line L427 (19.4801, 50.2361) -> (17.8105, 49.4915) construction
  line L428 (17.8105, 49.4915) -> (16.8249, 49.2742) construction
  line L429 (16.8249, 49.2742) -> (15.9023, 48.953) construction
  line L430 (15.9023, 48.953) -> (15.081, 48.6521) construction
  line L431 (15.081, 48.6521) -> (14.2641, 48.1892) construction
  line L432 (14.2641, 48.1892) -> (13.8247, 48.1892) construction
  line L433 (13.8247, 48.1892) -> (13.3491, 48.0113) construction
  line L434 (13.3491, 48.0113) -> (12.9105, 47.6947) construction
  line L435 (12.9105, 47.6947) -> (12.7465, 47.9428) construction
  line L436 (12.7465, 47.9428) -> (12.7465, 48.202) construction
  line L437 (12.7465, 48.202) -> (13.048, 48.479) construction
  line L438 (13.048, 48.479) -> (13.8758, 48.948) construction
  line L439 (13.8758, 48.948) -> (14.996, 49.7866) construction
  line L440 (14.996, 49.7866) -> (16.524, 50.832) construction
  line L441 (16.524, 50.832) -> (17.8174, 51.6615) construction
  line L442 (17.8174, 51.6615) -> (19.6472, 52.8827) construction
  line L443 (19.6472, 52.8827) -> (22.6023, 54.9106) construction
  line L444 (22.6023, 54.9106) -> (25.0704, 56.3719) construction
  line L445 (25.0704, 56.3719) -> (27.3371, 57.7137) construction
  line L446 (27.3371, 57.7137) -> (30.3003, 59.3455) construction
  line L447 (30.3003, 59.3455) -> (33.7762, 61.0497) construction
  line L448 (33.7762, 61.0497) -> (36.6162, 62.2885) construction
  line L449 (36.6162, 62.2885) -> (37.7754, 62.9631) construction
  line L450 (37.7754, 62.9631) -> (38.1447, 63.2072) construction
  line L451 (38.1447, 63.2072) -> (38.3811, 63.2072) construction
  line L452 (38.3811, 63.2072) -> (38.692, 62.9723) construction
  line L453 (38.692, 62.9723) -> (39.0576, 62.4087) construction
  line L454 (39.0576, 62.4087) -> (39.3575, 61.6079) construction
  line L455 (39.3575, 61.6079) -> (39.6336, 60.7939) construction
  line L456 (39.6336, 60.7939) -> (39.8746, 59.9569) construction
  spline S12 degree 4 poles (54.9007, 54.8596) (54.4765, 54.7136) (53.9435, 54.7136) (52.7301, 54.7136) (51.4894, 54.7136) (49.6881, 54.7136) (47.5629, 54.8596) (45.9313, 55.1419) (43.8712, 55.2718) (43.2767, 55.3696) (42.8621, 55.6655) (41.1619, 56.0816) (40.5893, 56.292) (39.9821, 56.292) (39.2171, 56.292) (38.4402, 56.0817) (37.6861, 55.8637) (36.3853, 55.5789) (36.1116, 55.3696) (35.3358, 55.1419) (34.2482, 54.9037) (32.1688, 54.4484) (30.0993, 53.784) (28.8674, 53.4238) (27.2155, 52.8935) (25.7568, 52.4669) (23.2013, 51.5305) (21.9891, 51.1414) (20.9902, 50.832) (19.4801, 50.2361) (17.8105, 49.4915) (16.8249, 49.2742) (15.9023, 48.953) (15.081, 48.6521) (14.2641, 48.1892) (13.8247, 48.1892) (13.3491, 48.0113) (12.9105, 47.6947) (12.7465, 47.9428) (12.7465, 48.202) (13.048, 48.479) (13.8758, 48.948) (14.996, 49.7866) (16.524, 50.832) (17.8174, 51.6615) (19.6472, 52.8827) (22.6023, 54.9106) (25.0704, 56.3719) (27.3371, 57.7137) (30.3003, 59.3455) (33.7762, 61.0497) (36.6162, 62.2885) (37.7754, 62.9631) (38.1447, 63.2072) (38.3811, 63.2072) (38.692, 62.9723) (39.0576, 62.4087) (39.3575, 61.6079) (39.6336, 60.7939) (39.8746, 59.9569) knots 1 1 1 1 1 2 3 4 5 6 7 8 9 10 11 12 13 14 15 16 17 18 19 20 21 22 23 24 25 26 27 28 29 30 31 32 33 34 35 36 37 38 39 40 41 42 43 44 45 46 47 48 49 50 51 52 53 54 55 56 57 57 57 57 57
  line L457 (42.4975, 61.486) -> (42.0758, 61.9752) construction
  line L458 (42.0758, 61.9752) -> (42.0758, 62.1342) construction
  line L459 (42.0758, 62.1342) -> (42.5548, 61.8855) construction
  line L460 (42.5548, 61.8855) -> (44.0577, 60.76) construction
  line L461 (44.0577, 60.76) -> (46.2308, 59.509) construction
  line L462 (46.2308, 59.509) -> (47.4843, 58.5296) construction
  line L463 (47.4843, 58.5296) -> (48.2148, 58.006) construction
  line L464 (48.2148, 58.006) -> (48.3603, 57.7029) construction
  spline S13 degree 4 poles (42.4975, 61.486) (42.0758, 61.9752) (42.0758, 62.1342) (42.5548, 61.8855) (44.0577, 60.76) (46.2308, 59.509) (47.4843, 58.5296) (48.2148, 58.006) (48.3603, 57.7029) knots 1 1 1 1 1 2 3 4 5 6 6 6 6 6
  line L465 (49.6634, 60.0271) -> (49.455, 60.1955) construction
  line L466 (49.455, 60.1955) -> (50.2498, 60.303) construction
  line L467 (50.2498, 60.303) -> (52.6013, 60.2516) construction
  line L468 (52.6013, 60.2516) -> (53.624, 60.2709) construction
  line L469 (53.624, 60.2709) -> (54.9938, 60.263) construction
  line L470 (54.9938, 60.263) -> (55.6985, 60.1997) construction
  spline S14 degree 4 poles (49.6634, 60.0271) (49.455, 60.1955) (50.2498, 60.303) (52.6013, 60.2516) (53.624, 60.2709) (54.9938, 60.263) (55.6985, 60.1997) knots 1 1 1 1 1 2 3 4 4 4 4 4
  line L471 (57.9839, 62.4087) -> (58.4584, 62.7299) construction
  line L472 (58.4584, 62.7299) -> (59.4882, 63.4429) construction
  line L473 (59.4882, 63.4429) -> (60.9446, 64.2107) construction
  line L474 (60.9446, 64.2107) -> (61.7063, 64.6129) construction
  line L475 (61.7063, 64.6129) -> (62.5133, 65.3895) construction
  line L476 (62.5133, 65.3895) -> (62.3275, 65.823) construction
  line L477 (62.3275, 65.823) -> (61.9353, 66.2564) construction
  line L478 (61.9353, 66.2564) -> (60.7175, 67.0718) construction
  line L479 (60.7175, 67.0718) -> (59.3035, 67.722) construction
  line L480 (59.3035, 67.722) -> (58.2302, 68.1348) construction
  line L481 (58.2302, 68.1348) -> (56.2589, 68.5064) construction
  line L482 (56.2589, 68.5064) -> (54.8489, 68.7892) construction
  line L483 (54.8489, 68.7892) -> (52.961, 68.8067) construction
  line L484 (52.961, 68.8067) -> (50.0244, 68.7892) construction
  line L485 (50.0244, 68.7892) -> (48.6435, 68.6144) construction
  line L486 (48.6435, 68.6144) -> (47.8219, 68.2124) construction
  line L487 (47.8219, 68.2124) -> (46.843, 68.0376) construction
  line L488 (46.843, 68.0376) -> (46.3186, 67.8628) construction
  line L489 (46.3186, 67.8628) -> (45.8621, 67.8078) construction
  spline S15 degree 4 poles (57.9839, 62.4087) (58.4584, 62.7299) (59.4882, 63.4429) (60.9446, 64.2107) (61.7063, 64.6129) (62.5133, 65.3895) (62.3275, 65.823) (61.9353, 66.2564) (60.7175, 67.0718) (59.3035, 67.722) (58.2302, 68.1348) (56.2589, 68.5064) (54.8489, 68.7892) (52.961, 68.8067) (50.0244, 68.7892) (48.6435, 68.6144) (47.8219, 68.2124) (46.843, 68.0376) (46.3186, 67.8628) (45.8621, 67.8078) knots 1 1 1 1 1 2 3 4 5 6 7 8 9 10 11 12 13 14 15 16 17 17 17 17 17
  line L490 (45.6531, 65.823) -> (46.3391, 65.3329) construction
  line L491 (46.3391, 65.3329) -> (47.363, 64.7155) construction
  line L492 (47.363, 64.7155) -> (46.9113, 64.7155) construction
  line L493 (46.9113, 64.7155) -> (46.1735, 64.7456) construction
  line L494 (46.1735, 64.7456) -> (45.526, 64.8058) construction
  line L495 (45.526, 64.8058) -> (44.9796, 65.3895) construction
  spline S16 degree 4 poles (45.6531, 65.823) (46.3391, 65.3329) (47.363, 64.7155) (46.9113, 64.7155) (46.1735, 64.7456) (45.526, 64.8058) (44.9796, 65.3895) knots 1 1 1 1 1 2 3 4 4 4 4 4
  line L496 (43.1549, 65.9285) -> (42.5597, 65.905) construction
  line L497 (42.5597, 65.905) -> (41.6412, 66.2815) construction
  line L498 (41.6412, 66.2815) -> (40.3764, 66.8085) construction
  line L499 (40.3764, 66.8085) -> (39.3525, 67.4559) construction
  line L500 (39.3525, 67.4559) -> (38.6599, 67.8474) construction
  line L501 (38.6599, 67.8474) -> (38.8556, 68.013) construction
  line L502 (38.8556, 68.013) -> (40.2409, 67.9528) construction
  line L503 (40.2409, 67.9528) -> (41.7767, 67.8926) construction
  line L504 (41.7767, 67.8926) -> (43.3818, 68.2124) construction
  spline S17 degree 4 poles (43.1549, 65.9285) (42.5597, 65.905) (41.6412, 66.2815) (40.3764, 66.8085) (39.3525, 67.4559) (38.6599, 67.8474) (38.8556, 68.013) (40.2409, 67.9528) (41.7767, 67.8926) (43.3818, 68.2124) knots 1 1 1 1 1 2 3 4 5 6 7 7 7 7 7
  line L505 (44.9532, 68.5254) -> (45.8572, 68.5551) construction
  line L506 (45.8572, 68.5551) -> (46.3993, 68.9466) construction
  line L507 (46.3993, 68.9466) -> (48.5826, 69.6995) construction
  line L508 (48.5826, 69.6995) -> (50.0733, 70.1361) construction
  line L509 (50.0733, 70.1361) -> (52.0608, 70.5126) construction
  line L510 (52.0608, 70.5126) -> (53.943, 70.5276) construction
  line L511 (53.943, 70.5276) -> (55.9005, 70.2566) construction
  line L512 (55.9005, 70.2566) -> (58.415, 69.7597) construction
  line L513 (58.415, 69.7597) -> (59.454, 69.579) construction
  line L514 (59.454, 69.579) -> (61.1404, 68.9165) construction
  line L515 (61.1404, 68.9165) -> (62.0288, 68.0733) construction
  line L516 (62.0288, 68.0733) -> (62.2715, 67.6288) construction
  spline S18 degree 4 poles (44.9532, 68.5254) (45.8572, 68.5551) (46.3993, 68.9466) (48.5826, 69.6995) (50.0733, 70.1361) (52.0608, 70.5126) (53.943, 70.5276) (55.9005, 70.2566) (58.415, 69.7597) (59.454, 69.579) (61.1404, 68.9165) (62.0288, 68.0733) (62.2715, 67.6288) knots 1 1 1 1 1 2 3 4 5 6 7 8 9 10 10 10 10 10
  line L517 (63.2685, 70.0081) -> (62.9924, 70.1512) construction
  line L518 (62.9924, 70.1512) -> (62.9774, 70.3018) construction
  line L519 (62.9774, 70.3018) -> (63.4893, 70.4674) construction
  line L520 (63.4893, 70.4674) -> (66.6514, 70.9944) construction
  line L521 (66.6514, 70.9944) -> (71.9063, 71.3106) construction
  line L522 (71.9063, 71.3106) -> (74.9329, 71.4009) construction
  line L523 (74.9329, 71.4009) -> (78.0798, 71.4009) construction
  line L524 (78.0798, 71.4009) -> (79.706, 71.3859) construction
  line L525 (79.706, 71.3859) -> (80.218, 71.3859) construction
  line L526 (80.218, 71.3859) -> (80.6245, 70.9643) construction
  line L527 (80.6245, 70.9643) -> (81.1365, 70.1662) construction
  line L528 (81.1365, 70.1662) -> (81.5129, 69.5639) construction
  line L529 (81.5129, 69.5639) -> (81.5975, 68.8428) construction